headphone_holder (Autodesk Fusion 360 design; units mm, degrees)
Autodesk Fusion 360 part; units mm, degrees
sketch "Sketch1" plane through (0, 0, 0) normal (0, 1, 0) x (1, 0, 0)
  line L0 (0, 0) -> (-90, 0)
  line L1 (-90, 0) -> (-90, -8)
  line L2 (-90, -8) -> (0, -8)
  line L3 (0, -8) -> (0, 0)
  arc A0 (-90, 0) -> (0, 0) centre (-45, 122.5625) ccw
  line L4 (-90, 0) -> (0, 0)
  line L5 (0, 0) -> (0, 1.5)
  line L6 (0, 1.5) -> (-90, 1.5)
  line L7 (-90, 1.5) -> (-90, 0)
  arc A1 (-90, 1.5) -> (0, 1.5) centre (-45, 287.9873) ccw
  dimension "d1" = 8
  dimension "d2" = 90
  dimension "d3" = 1.5
  dimension "d4" = 290
  constraint horizontal L0
  constraint vertical L1
  constraint horizontal L2
  constraint vertical L3
  constraint coincident L0.start L3.end
  constraint tangent L2 A0
  constraint horizontal L4
  constraint vertical L5
  constraint horizontal L6
  constraint vertical L7
  measures "d1" distance of L0.start L2.end
  measures "d2" distance of L1.end L2.end
  measures "d3" distance of L0.end L6.end
  measures "d4" radius of A1
extrude "Extrude1" add sketch "Sketch1" along normal blind 40 contours L0 A0 L4 A1 | L0 L4 L5 A1 | L0 L4 L7 A1
sketch "Sketch2" plane through (0, 40, 0) normal (0, 1, 0) x (-1, 0, 0)
  arc A0 (90, 0) -> (0, 0) centre (45, -122.5625) ccw
  line L0 (0, 0) -> (0, -1.5)
  arc A1 (90, -1.5) -> (0, -1.5) centre (45, -287.9873) ccw
  line L1 (90, -1.5) -> (90, 0)
  line L2 (90, -1.5) -> (45, -35.4099)
  line L3 (45, -35.4099) -> (0, -1.5)
  line L4 (83.0298, -0.4917) -> (45, -29.1493)
  line L5 (45, -29.1493) -> (6.9702, -0.4917)
  line L6 (45, -35.4099) -> (45, 3)
  line L7 (55, -21.6137) -> (55, 1.8402)
  line L8 (55, 1.8402) -> (45, 3)
  line L9 (45, 3) -> (35, 1.8402)
  line L10 (59.0023, 1.6744) -> (68.7457, -11.2556)
  line L11 (6.9702, -0.4917) -> (83.0298, -0.4917)
  line L12 (55, -0.4917) -> (65.1519, -13.9637)
  line L13 (30.9977, 1.6744) -> (21.2543, -11.2556)
  line L14 (35, -0.4917) -> (24.8481, -13.9637)
  line L15 (35, -21.6137) -> (35, 1.8402)
  dimension "d8" = 10
  dimension "d9" = 5
  dimension "d10" = 5
  dimension "d13" = 37
  dimension "d14" = 90
  dimension "d15" = 4.5
  constraint coincident A1.start L1.start
  constraint coincident L0.end A1.end
  constraint coincident A1 L4.start
  constraint parallel L2 L4
  constraint coincident A1 L5.end
  constraint parallel L3 L5
  constraint vertical L6
  constraint coincident L4 L7.start
  constraint coincident A1 L7.end
  constraint vertical L7
  constraint coincident A1 L9.end
  constraint coincident A1 L10.start
  constraint coincident L4 L10.end
  constraint horizontal L11
  constraint coincident L7 L12.start
  constraint coincident L11 L12.start
  constraint coincident L4 L12.end
  constraint perpendicular L4 L12
  constraint symmetric L6 L7.start L15.start
  constraint symmetric L6 L7.end L9.end
  constraint symmetric L6 L10.start L13.start
  constraint symmetric L6 L10.end L13.end
  constraint symmetric L6 L12.start L14.start
  constraint symmetric L6 L12.end L14.end
  measures "d8" distance of L6 L7
  measures "d9" distance of L2 L4
  measures "d10" distance of L3 L5
  measures "d13" angle of L4 L11
  measures "d14" angle of L4 L10
  measures "d15" distance of L10 L12
extrude "Extrude2" add sketch "Sketch2" against normal blind 4 contours A1 L2 L4 L6 | A1 L3 L5 L6 | A1 L7 L10 L11 | L4 L10 L11 L12 | L4 L6 L7 L11 | L5 L6 L11 L15 | A1 L11 L13 L15 | L5 L11 L13 L14 | A1 L6 L7 L11 | A1 L6 L11 L15
ref_plane "WorkPlane1" through (-45, 0, 0) normal (1, 0, 0) x (0, 1, 0)
sketch "Sketch3" plane through (-45, 0, 0) normal (1, 0, 0) x (0, 1, 0)
  line L0 (17, 3) -> (36, -24)
  line L1 (36, -24) -> (36, -18.7871)
  line L2 (36, -18.7871) -> (20.2674, 3.5698)
  line L3 (20.2674, 3.5698) -> (17, 3)
  dimension "d17" = 3
  constraint vertical L1
  constraint parallel L0 L2
  measures "d17" distance of L0 L2
extrude "Extrude3" add sketch "Sketch3" along normal mid plane 6
